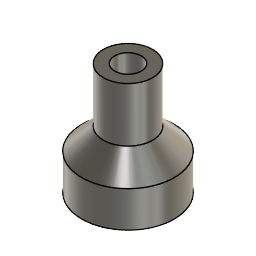
MagnetStandoff_v1 (Autodesk Fusion 360 design; units mm, degrees)
Autodesk Fusion 360 part; units mm, degrees
sketch "Sketch1" plane through (0, 0, 0) normal (0, 0, 1) x (1, 0, 0)
  circle A0 centre (0, 0) radius 1.75
  circle A1 centre (0, 0) radius 3.25
  circle A2 centre (0, 0) radius 5.1
  circle A3 centre (0, 0) radius 6.1
  dimension "d1" = 3.5
  dimension "d2" = 1.5
  dimension "d7" = 10.2
  dimension "d8" = 1
  constraint coincident A0.centre A1.centre
  constraint concentric A1 A2
  constraint concentric A2 A3
  measures "d1" diameter of A0
  measures "d2" distance of A0 A1
  measures "d7" diameter of A2
  measures "d8" distance of A2 A3
extrude "Extrude1" add sketch "Sketch1" along normal blind 6 contours A1
extrude "Extrude2" add sketch "Sketch1" against normal blind 6 contours A0 | A1
extrude "Extrude3" add sketch "Sketch1" against normal blind 2 from surface at -4 contours A2 | A3
extrude "Extrude4" add sketch "Sketch1" against normal blind 2.75 from surface at -6 contours A3
chamfer "Chamfer1" distance 2.85 angle 45 1 edges at (-3.0301, -1.1753, -4) tangent chain off
